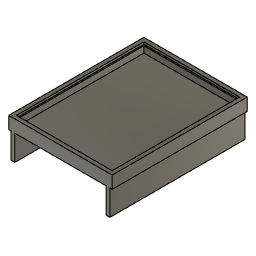
driver_board_holder (Autodesk Fusion 360 design; units mm, degrees)
Autodesk Fusion 360 part; units mm, degrees
note: some values were not read from the file. Set by a fixed rule: which sketch regions a step uses.
sketch "Sketch1" plane through (0, 0, 0) normal (0, 0, 1) x (1, 0, 0)
  line L0 (0, 0) -> (3, 0)
  line L1 (3, 0) -> (3, 106.5)
  line L2 (3, 106.5) -> (0, 106.5)
  line L3 (0, 106.5) -> (0, 0)
  line L4 (75, 0) -> (78, 0)
  line L5 (78, 0) -> (78, 106.5)
  line L6 (78, 106.5) -> (75, 106.5)
  line L7 (75, 106.5) -> (75, 0)
  dimension "d8" = 3
  dimension "d9" = 106.5
  dimension "d10" = 3
  dimension "d11" = 106.5
  dimension "d12" = 72
  constraint horizontal L0
  constraint vertical L1
  constraint horizontal L2
  constraint vertical L3
  constraint coincident L0.start L3.end
  constraint horizontal L4
  constraint vertical L5
  constraint horizontal L6
  constraint vertical L7
  measures "d8" distance of L0.start L0.end
  measures "d9" distance of L0.start L2.end
  measures "d10" distance of L4.start L4.end
  measures "d11" distance of L4.start L6.end
  measures "d12" distance of L1 L7
extrude "Extrude1" add sketch "Sketch1" along normal blind 20 makes body 1 at (75, 71, 13.3333) makes body 2 at (0, 71, 13.3333)
sketch "Sketch2" plane through (0, 0, 20) normal (0, 0, 1) x (-1, 0, 0)
  line L0 (0, -106.5) -> (0, 0)
  line L1 (0, 0) -> (-3, 0)
  line L2 (-3, 0) -> (-3, -106.5)
  line L3 (-3, -106.5) -> (0, -106.5)
  line L4 (0, 0) -> (-78, 0) construction
  line L5 (-39, 0) -> (1.75, 0) construction
  line L6 (-39, 0) -> (-79.75, 0) construction
  line L7 (-79.75, 0) -> (1.75, 0)
  line L8 (-79.75, 0) -> (1.75, 0)
  line L9 (1.75, 0) -> (1.75, -106.5)
  line L10 (1.75, -106.5) -> (-79.75, -106.5)
  line L11 (-79.75, -106.5) -> (-79.75, 0)
  dimension "d15" = 40.75
  dimension "d16" = 40.75
  dimension "d27" = 81.5
  dimension "d28" = 106.5
  constraint coincident L0.end L1.start
  constraint perpendicular L0 L4
  constraint midpoint L4 L5.start
  constraint perpendicular L0 L5
  constraint parallel L4 L6
  constraint horizontal L7
  constraint horizontal L8
  constraint vertical L9
  constraint horizontal L10
  constraint vertical L11
  measures "d15" distance of L5.start L5.end
  measures "d16" distance of L5.start L6.end
  measures "d27" distance of L6.end L5.end
  measures "d28" distance of L6.end L10.end
extrude "Extrude2" add sketch "Sketch2" along normal blind 3 bodies 1 2
sketch "Sketch3" plane through (0, 0, 23) normal (0, 0, 1) x (-1, 0, 0)
  line L0 (-79.75, -106.5) -> (1.75, -106.5)
  line L1 (1.75, 0) -> (-79.75, 0)
  line L2 (1.75, -106.5) -> (1.75, 0)
  line L3 (-79.75, 0) -> (-79.75, -106.5)
  line L4 (-76.75, -3) -> (-76.75, -103.5)
  line L5 (-76.75, -103.5) -> (-1.25, -103.5)
  line L6 (-1.25, -103.5) -> (-1.25, -3)
  line L7 (-1.25, -3) -> (-76.75, -3)
extrude "Extrude3" add sketch "Sketch3" along normal blind 6.75 bodies 1
sketch "Sketch4" plane through (0, 0, 23) normal (0, 0, 1) x (-1, 0, 0)
  line L0 (-76.75, -3) -> (-76.75, -103.5)
  line L1 (-76.75, -103.5) -> (-1.25, -103.5)
  line L2 (-1.25, -103.5) -> (-1.25, -3)
  line L3 (-1.25, -3) -> (-76.75, -3)
  line L4 (-2.25, -4) -> (-75.75, -4)
  line L5 (-75.75, -4) -> (-75.75, -102.5)
  line L6 (-75.75, -102.5) -> (-2.25, -102.5)
  line L7 (-2.25, -102.5) -> (-2.25, -4)
extrude "Extrude4" add sketch "Sketch4" along normal blind 5 bodies 1
equation "thickness = 3 mm"
equation "bottom_gap = 72 mm"
equation "board_width = 75 mm"
equation "board_length = 100 mm"
equation "tolerance = 0.25 mm"
equation "height_under_board = 5 mm"
equation "bottom_height = 20 mm"
equation "d8 = thickness"
equation "d9 = board_length + thickness * 2 + tolerance * 2"
equation "d10 = thickness"
equation "d11 = board_length + thickness * 2 + tolerance * 2"
equation "d12 = bottom_gap"
equation "d15 = board_width / 2 + thickness + tolerance"
equation "d16 = board_width / 2 + thickness + tolerance"
equation "d17 = thickness"
equation "board_thickness = 1.75 mm"
equation "d21 = height_under_board + board_thickness"
equation "board_lip = 1 mm"
equation "d25 = height_under_board"
equation "d27 = board_width + tolerance * 2 + thickness * 2"
equation "d28 = board_length + tolerance * 2 + thickness * 2"
equation "d29 = -thickness"
equation "d30 = -board_lip"
